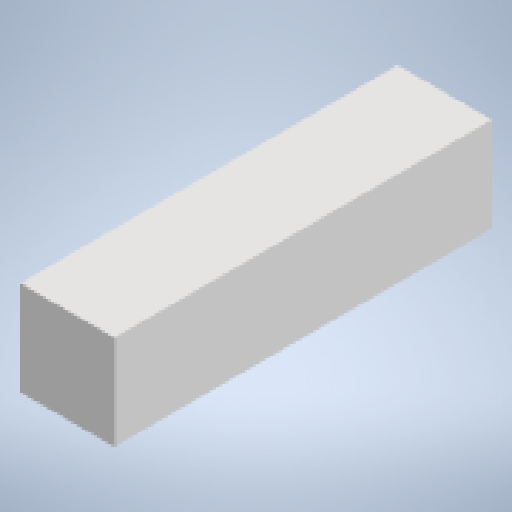
# Autodesk Inventor part: Max_Payload
Saved by Autodesk Inventor 2027.1 (Build 311270010, 270A)
## iProperties
Created: 2026-09-09
Part Number: Max_Payload
Material: Generic
Document SubType Name: Modeling
Designer: PWYNNE
Density: 0.72338 g/cm^3
Appearance: Default
Mass: 5000 g
Surface Area: 2592 cm^2
Volume: 6912 cm^3
Author: PWYNNE
Autodesk Inventor part; units mm, degrees
ref_plane "YZ Plane" through (0, 0, 0) normal (1, 0, 0) x (0, 1, 0)
ref_plane "XZ Plane" through (0, 0, 0) normal (0, 1, 0) x (-1, 0, 0)
ref_plane "XY Plane" through (0, 0, 0) normal (0, 0, 1) x (1, 0, 0)
sketch "Sketch1" plane through (0, 0, 0) normal (0, 1, 0) x (-1, 0, 0)
  line L0 (-60, 240) -> (60, 240)
  line L1 (60, 240) -> (60, -240)
  line L2 (60, -240) -> (-60, -240)
  line L3 (-60, -240) -> (-60, 240)
  line L4 (-60, 240) -> (60, -240) construction
  line L5 (60, 240) -> (-60, -240) construction
  point P0 (0, 0)
  dimension "d0" = 480
  dimension "d1" = 120
  constraints: 12 end point, 2 midpoint, 2 parallel, 1 horizontal, 1 perpendicular
  measures "d0" distance of L0.end L1.end
  measures "d1" distance of L1.end L2.end
extrude "Extrusion1" add sketch "Sketch1" along normal blind 120
body "Solid1"
